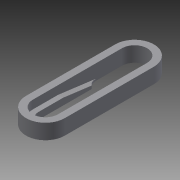
# Autodesk Inventor part: bed-holder-b
Saved by Autodesk Inventor 2015 (Build 190159000, 159)
## iProperties
Created: 2014-10-22
Part Number: bed-holder-b
Material: Generic
Document SubType Name: Modeling
Designer: caleb
Density: 1 g/cm^3
Appearance: Default
Author: caleb
Autodesk Inventor part; units mm, degrees
ref_plane "YZ Plane" through (0, 0, 0) normal (1, 0, 0) x (0, 1, 0)
ref_plane "XZ Plane" through (0, 0, 0) normal (0, 1, 0) x (-1, 0, 0)
ref_plane "XY Plane" through (0, 0, 0) normal (0, 0, 1) x (1, 0, 0)
sketch "Sketch6" plane through (0, 0, 0) normal (0, 0, 1) x (1, 0, 0)
  line L0 (0, 0) -> (0, -26.5) construction
  line L1 (-3.75, 0) -> (-3.75, -26.5)
  line L2 (3.75, -26.5) -> (3.75, 0)
  arc A0 (3.75, 0) -> (-3.75, 0) centre (0, 0) ccw
  arc A1 (-3.75, -26.5) -> (3.75, -26.5) centre (0, -26.5) ccw
  line L3 (5.75, 0) -> (5.75, -26.5)
  arc A2 (-5.75, -26.5) -> (5.75, -26.5) centre (0, -26.5) ccw
  line L4 (-5.75, -26.5) -> (-5.75, 0)
  arc A3 (5.75, 0) -> (-5.75, 0) centre (0, 0) ccw
  line L5 (0, 5.75) -> (0, -32.25) construction
  line L6 (0, 0) -> (0, -26.5) construction
  line L7 (-2.25, 0) -> (-2.25, -3)
  line L8 (2.25, -26.5) -> (2.25, -3)
  arc A4 (2.25, 0) -> (-2.25, 0) centre (0, 0) ccw
  arc A5 (-2.25, -26.5) -> (2.25, -26.5) centre (0, -26.5) ccw
  arc A6 (-3.75, 0) -> (3.75, 0) centre (0, 0) ccw
  line L9 (-2.25, -3) -> (-2.25, -26.5)
  line L10 (2.25, -3) -> (2.25, 0)
  point P0 (0, -13.25)
  point P1 (0, -13.25)
  dimension "d20" = 3.75
  dimension "d21" = 2
  dimension "d23" = 4.5
  dimension "d33" = 38
  constraints: 26 end point, 18 point on circle, 13 tangent, 7 centre point, 6 parallel, 2 midpoint, 1 collinear, 1 vertical, 3 other
  measures "d20" radius of A0
  measures "d21" distance between parallel lines of L3 L2
  measures "d23" distance between parallel lines of L8 L7
  measures "d33" distance of L5.start L5.end
extrude "Extrusion7" add sketch "Sketch6" along normal blind 4.5
sketch "Sketch7" plane through (0, 0, 0) normal (1, 0, 0) x (0, 1, 0)
  line L0 (-7.5, 0.5) -> (-19, 2) construction
  line L1 (-19, 2) -> (-19, 0) construction
  point P0 (0, 0)
  point P1 (-26.5, 0)
  dimension "d28" = 7.5
  dimension "d29" = 2
  dimension "d34" = 0.5
  dimension "d35" = 7.5
  constraints: 4 end point, 1 horizontal alignment, 1 vertical
  measures "d28" horizontal distance of point (-26.5, 0) L0.end
  measures "d29" vertical distance of L0.end point (-26.5, 0)
  measures "d34" vertical distance of L0.start point (0, 0)
  measures "d35" horizontal distance of L0.start point (0, 0)
ref_plane "Work Plane3" through (0, -7.5, 0.5) normal (0, 0.1293392, 0.9916004) x (0, -0.9916004, 0.1293392)
extrude "Extrusion9" add sketch "Sketch6" along normal blind 2 separate body contours A6 L9 A5 L8 L2 A1 L1
split "Split1" plane through (0, -7.5, 0.5) removes the side toward (0, 0.1293392, 0.9916004) bodies 2
combine bodies "Combine1" operation type add bodies to combine 1 2
sketch "Sketch8" plane through (0, -26.5, 0) normal (0, 0, -1) x (-1, 0, 0)
  line L0 (0, 26.5) -> (0, 19) construction
  line L1 (-3.75, 26.5) -> (-3.75, 19)
  line L2 (3.75, 19) -> (3.75, 26.5)
  arc A0 (3.75, 26.5) -> (-3.75, 26.5) centre (0, 26.5) ccw
  arc A1 (-3.75, 19) -> (3.75, 19) centre (0, 19) ccw
  arc A2 (3.75, 26.5) -> (-3.75, 26.5) centre (0, 26.5) ccw projected
  point P0 (0, 22.75)
  dimension "d36" = 7.5
  constraints: 8 end point, 4 point on circle, 4 tangent, 2 centre point, 1 concentric, 1 midpoint, 1 parallel, 1 vertical
  measures "d36" distance of L0.start L0.end
extrude "Extrusion10" cut sketch "Sketch8" against normal through all bodies 1
equation "\"d20\" = 0.5 * screw_head_diameter_1"
equation "\"d21\" = wall_1"
equation "\"d23\" = screw_diameter_1"
equation "\"d33\" = length"
equation "\"d24\" = height_1"
equation "\"d28\" = screw_head_diameter_1"
equation "\"d29\" = land_height_1"
equation "\"d35\" = screw_head_diameter_1"
equation "\"d31\" = land_height_1"
equation "\"d36\" = screw_head_diameter_1"
equation "\"screw_head_diameter_1\" = 7.5"
equation "\"wall_1\" = 2"
equation "\"screw_diameter_1\" = 4.5"
equation "\"length\" = 38"
equation "\"height_1\" = 4.5"
equation "\"land_height_1\" = 2"
body "Solid2"
